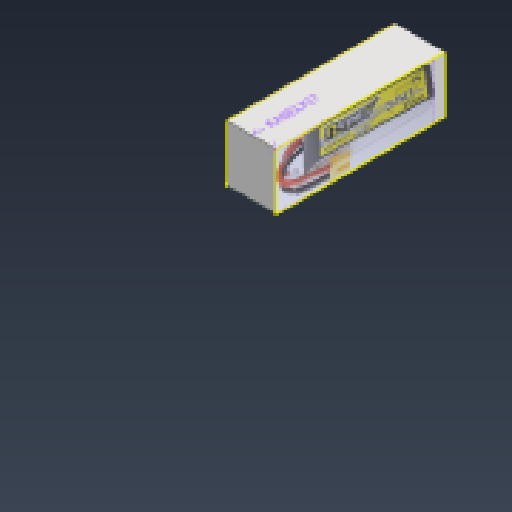
# Autodesk Inventor part: lipo-3s-550mah
Saved by Autodesk Inventor 2023 (Build 270158000, 158)
## iProperties
Created: 2025-03-29
Part Number: lipo-3s-550mah
Material: Generic
Document SubType Name: Modeling
Designer: szymo
Density: 1 g/cm^3
Appearance: Default
Author: szymo
Autodesk Inventor part; units mm, degrees
ref_plane "YZ Plane" through (0, 0, 0) normal (1, 0, 0) x (0, 1, 0)
ref_plane "XZ Plane" through (0, 0, 0) normal (0, 1, 0) x (-1, 0, 0)
ref_plane "XY Plane" through (0, 0, 0) normal (0, 0, 1) x (1, 0, 0)
sketch "Sketch1" plane through (0, 0, 0) normal (0, 1, 0) x (-1, 0, 0)
  line L0 (0, 0) -> (18.5, 0)
  line L1 (18.5, 0) -> (18.5, -63)
  line L2 (18.5, -63) -> (0, -63)
  line L3 (0, -63) -> (0, 0)
  dimension "d0" = 18.5
  dimension "d1" = 63
  constraints: 8 end point, 2 parallel, 1 horizontal, 1 perpendicular
  measures "d0" distance of L1.end L2.end
  measures "d1" distance of L0.end L1.end
extrude "Extrusion1" add sketch "Sketch1" along normal blind 21
sketch "Sketch2" plane through (0, 21, 0) normal (1, 0, 0) x (0, -1, 0)
  line L0 (21, 0) -> (21, 63) projected
  line L1 (21, 63) -> (0, 63) projected
  line L2 (0, 0) -> (0, 63) projected
  line L3 (21, 0) -> (0, 0) projected
  line L4 (21.019, -0.0304) -> (0, 0) construction
  line L5 (0, 0) -> (0.0859, 59.3529) construction
  line L6 (0.0859, 59.3529) -> (21.105, 59.3225) construction
  line L7 (21.105, 59.3225) -> (21.019, -0.0304) construction
  constraints: 1 coincident, 2 other
sketch "Sketch3" plane through (-18.5, 0, -63) normal (-1, 0, 0) x (0, 0, 1)
  line L0 (0, 0) -> (63, 0) projected
  line L1 (63, 0) -> (63, 21) projected
  line L2 (0, 21) -> (63, 21) projected
  line L3 (0, 0) -> (0, 21) projected
  line L4 (0.0214, -0.0604) -> (0, 21) construction
  line L5 (0, 21) -> (59.4697, 21.0604) construction
  line L6 (59.4697, 21.0604) -> (59.4911, 0) construction
  line L7 (59.4911, 0) -> (0.0214, -0.0604) construction
  constraints: 2 coincident, 1 point on line, 2 other
sketch "Sketch4" plane through (0, 21, 0) normal (0, 1, 0) x (1, 0, 0)
  line L0 (-18.4095, 0) -> (-18.4095, 63) construction
  line L1 (-18.4095, 63) -> (0, 63) construction
  line L2 (0, 63) -> (0, 0) construction
  line L3 (0, 0) -> (-18.4095, 0) construction
  line L4 (0, 0) -> (0, 63) projected
  constraints: 1 coincident, 1 collinear, 2 other
body "Solid1"
